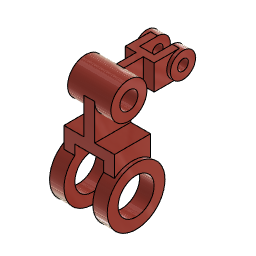
MAD 5 v1 (Autodesk Fusion 360 design; units mm, degrees)
Autodesk Fusion 360 part; units mm, degrees
sketch "Sketch1" plane through (0, 0, 0) normal (0, 1, 0) x (1, 0, 0)
  circle A0 centre (0, 0) radius 12.5
  circle A1 centre (0, 0) radius 25
  circle A2 centre (0, 110) radius 25
  circle A3 centre (0, 110) radius 40
  circle A4 centre (-80, 0) radius 7.5
  circle A5 centre (-80, 0) radius 17.5
  dimension "d1" = 25
  dimension "d2" = 50
  dimension "d3" = 50
  dimension "d4" = 80
  dimension "d5" = 15
  dimension "d6" = 35
  dimension "d7" = 110
  dimension "d8" = 80
  constraint coincident A0.centre A1.centre
  constraint concentric A2 A3
  constraint concentric A4 A5
  measures "d1" diameter of A0
  measures "d2" diameter of A1
  measures "d3" diameter of A2
  measures "d4" diameter of A3
  measures "d5" diameter of A4
  measures "d6" diameter of A5
  measures "d7" distance of A0.centre A2.centre
  measures "d8" distance of A0.centre A4.centre
sketch "Sketch2" plane through (0, 0, 0) normal (1, 0, 0) x (0, 1, 0)
  circle A0 centre (0, 0) radius 25
  circle A1 centre (0, 0) radius 40
  circle A2 centre (0, 110) radius 12.5
  circle A3 centre (0, 110) radius 25
  circle A4 centre (80, 110) radius 7.5
  circle A5 centre (80, 110) radius 17.5
  dimension "d19" = 50
  dimension "d20" = 80
  dimension "d21" = 25
  dimension "d22" = 50
  dimension "d23" = 15
  dimension "d24" = 35
  dimension "d25" = 110
  dimension "d26" = 80
  dimension "d27" = 110
  constraint coincident A0.centre A1.centre
  constraint concentric A0 A1
  constraint concentric A2 A3
  constraint concentric A4 A5
  measures "d19" diameter of A0
  measures "d20" diameter of A1
  measures "d21" diameter of A2
  measures "d22" diameter of A3
  measures "d23" diameter of A4
  measures "d24" diameter of A5
  measures "d25" distance of A0.centre A2.centre
  measures "d26" horizontal distance of A0.centre A4.centre
  measures "d27" vertical distance of A0.centre A4.centre
extrude "Extrude6" add sketch "Sketch2" against normal blind 20 from surface at -20 contours A1 makes body 1
extrude "Extrude7" add sketch "Sketch2" against normal blind 15 from surface at -10 separate body contours A5 makes body 2
extrude "Extrude8" add sketch "Sketch2" along normal mid plane 60 separate body contours A3 makes body 3
mirror "Mirror1" about plane through (0, 0, 0) normal (1, 0, 0) of bodies 2 1 makes body 4 at (33.3333, 39.9503, -1.9938) makes body 5 at (20, 97.413, 108.2576)
sketch "Sketch3" plane through (0, 0, 0) normal (0, 1, 0) x (1, 0, 0)
  line L0 (40, 0) -> (40, -40)
  line L1 (40, 40) -> (40, 0)
  line L2 (20, 0) -> (20, 40)
  line L3 (20, -40) -> (20, 0)
  line L4 (40, 40) -> (20, 40)
  line L5 (40, -40) -> (20, -40)
  line L6 (-40, 0) -> (-40, -40)
  line L7 (-40, 40) -> (-40, 0)
  line L8 (-20, 0) -> (-20, 40)
  line L9 (-20, -40) -> (-20, 0)
  line L10 (-20, 40) -> (-40, 40)
  line L11 (-20, -40) -> (-40, -40)
  line L12 (-30, -110) -> (-30, -135)
  line L13 (-30, -85) -> (-30, -110)
  line L14 (30, -110) -> (30, -85)
  line L15 (30, -135) -> (30, -110)
  line L16 (-30, -135) -> (30, -135)
  line L17 (-30, -85) -> (30, -85)
  line L18 (-20, 0) -> (-35, 0)
  line L19 (-35, 0) -> (-35, -45)
  line L20 (-35, -45) -> (-20, -45)
  line L21 (-20, -45) -> (-20, 0)
  line L22 (20, 0) -> (35, 0)
  line L23 (35, 0) -> (35, -45)
  line L24 (35, -45) -> (20, -45)
  line L25 (20, -45) -> (20, 0)
  line L26 (35, -45) -> (-35, -45)
  line L27 (-35, -45) -> (-35, -60)
  line L28 (-35, -60) -> (35, -60)
  line L29 (35, -60) -> (35, -45)
  line L30 (7.5, -45) -> (-7.5, -45)
  line L31 (-7.5, -45) -> (-7.5, -110)
  line L32 (-7.5, -110) -> (7.5, -110)
  line L33 (7.5, -110) -> (7.5, -45)
  dimension "d38" = 15
  dimension "d39" = 45
  dimension "d40" = 15
  dimension "d41" = 45
  dimension "d42" = 15
  dimension "d43" = 15
  dimension "d44" = 65
  dimension "d45" = 27.5
  constraint horizontal L18
  constraint vertical L19
  constraint horizontal L20
  constraint vertical L21
  constraint coincident L8.start L9.end
  constraint horizontal L22
  constraint vertical L23
  constraint horizontal L24
  constraint vertical L25
  constraint coincident L2.start L3.end
  constraint horizontal L26
  constraint vertical L27
  constraint horizontal L28
  constraint vertical L29
  constraint horizontal L30
  constraint vertical L31
  constraint horizontal L32
  constraint vertical L33
  constraint coincident L26 L30.start
  constraint collinear L19 L27
  measures "d38" distance of L8.start L18.end
  measures "d39" distance of L8.start L20.end
  measures "d40" distance of L2.start L22.end
  measures "d41" distance of L2.start L24.end
  measures "d42" distance of L23.end L28.end
  measures "d43" distance of L30.start L30.end
  measures "d44" distance of L30.start L32.end
  measures "d45" distance of L27 L31
extrude "Extrude9" add sketch "Sketch3" along normal mid plane 50 separate body contours L5 L23 L24 L25 L26 | L3 L5 L22 L23 L25 | L24 L26 L28 L29 L33 | L26 L28 L30 L31 L33 | L17 L28 L31 L33 | L20 L26 L27 L28 L31 | L17 L31 L32 L33 | L11 L19 L20 L21 L26 | L9 L11 L18 L19 L21 makes body 6
extrude "Extrude10" cut sketch "Sketch2" along normal through all and the other way through all contours A0 | A2 bodies 6
ref_plane "WorkPlane1" through (-17.5, 80, 110) normal (0, 0, -1) x (-1, 0, 0)
sketch "Sketch4" plane through (0, 0, 110) normal (0, 0, -1) x (-1, 0, 0)
  line L0 (-25, 62.5) -> (-25, 97.5)
  line L1 (-10, 97.5) -> (-10, 62.5)
  line L2 (-25, 62.5) -> (-10, 62.5)
  line L3 (-25, 97.5) -> (-10, 97.5)
  line L4 (25, 62.5) -> (25, 97.5)
  line L5 (10, 97.5) -> (10, 62.5)
  line L6 (10, 62.5) -> (25, 62.5)
  line L7 (10, 97.5) -> (25, 97.5)
  line L8 (30, -25) -> (30, 25)
  line L9 (-30, 25) -> (-30, -25)
  line L10 (30, 25) -> (-30, 25)
  line L11 (30, -25) -> (-30, -25)
  line L12 (10, 80) -> (20, 80)
  line L13 (20, 80) -> (20, 55)
  line L14 (20, 55) -> (10, 55)
  line L15 (10, 55) -> (10, 80)
  line L16 (-10, 80) -> (-20, 80)
  line L17 (-20, 80) -> (-20, 55)
  line L18 (-20, 55) -> (-10, 55)
  line L19 (-10, 55) -> (-10, 80)
  line L20 (-20, 55) -> (20, 55)
  line L21 (20, 55) -> (20, 45)
  line L22 (20, 45) -> (-20, 45)
  line L23 (-20, 45) -> (-20, 55)
  line L24 (-5, 55) -> (5, 55)
  line L25 (5, 55) -> (5, 0)
  line L26 (5, 0) -> (-5, 0)
  line L27 (-5, 0) -> (-5, 55)
  dimension "d50" = 10
  dimension "d51" = 25
  dimension "d52" = 10
  dimension "d53" = 25
  dimension "d54" = 10
  dimension "d55" = 10
  dimension "d56" = 55
  dimension "d57" = 15
  dimension "d58" = 15
  constraint horizontal L12
  constraint vertical L13
  constraint horizontal L14
  constraint vertical L15
  constraint midpoint L5 L12.start
  constraint horizontal L16
  constraint vertical L17
  constraint horizontal L18
  constraint vertical L19
  constraint midpoint L1 L16.start
  constraint horizontal L20
  constraint vertical L21
  constraint horizontal L22
  constraint vertical L23
  constraint horizontal L24
  constraint vertical L25
  constraint horizontal L26
  constraint vertical L27
  constraint coincident L20 L24.start
  measures "d50" distance of L12.start L12.end
  measures "d51" distance of L12.start L14.end
  measures "d52" distance of L16.start L16.end
  measures "d53" distance of L16.start L18.end
  measures "d54" distance of L17.end L22.end
  measures "d55" distance of L24.start L24.end
  measures "d56" distance of L24.start L26.end
  measures "d57" distance of L21 L25
  measures "d58" distance of L23 L27
extrude "Extrude11" add sketch "Sketch4" along normal mid plane 35 separate body contours L1 L2 L16 L17 L19 | L2 L17 L18 L19 L20 | L18 L20 L22 L23 L27 | L20 L22 L24 L25 L27 | L10 L22 L25 L27 | L14 L20 L21 L22 L25 | L10 L25 L26 L27 | L6 L13 L14 L15 L20 | L5 L6 L12 L13 L15 makes body 7
extrude "Extrude12" cut sketch "Sketch2" along normal through all and the other way through all contours A2 | A4 bodies 7
combine "Combine1" operation add target body 3 tool bodies 6 7 2 5 1 4
